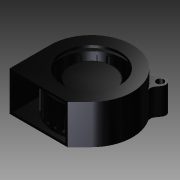
# Autodesk Inventor part: FanRadial40mm
Saved by Autodesk Inventor 2015 (Build 190159000, 159)
## iProperties
Created: 2014-12-06
Part Number: FanRadial40mm
Material: ABS Plastic
Document SubType Name: Modeling
Designer: Jack
Density: 1.06 g/cm^3
Appearance: Smooth - Black
Author: Jack
Autodesk Inventor part; units mm, degrees
ref_plane "YZ Plane" through (0, 0, 0) normal (1, 0, 0) x (0, 1, 0)
ref_plane "XZ Plane" through (0, 0, 0) normal (0, 1, 0) x (-1, 0, 0)
ref_plane "XY Plane" through (0, 0, 0) normal (0, 0, 1) x (1, 0, 0)
sketch "Sketch1" plane through (0, 0, 0) normal (0, 0, 1) x (1, 0, 0)
  arc A0 (14.2809, -14.002) -> (-20, 0) centre (0, 0) ccw
  line L0 (-20, 0) -> (-20, -20)
  line L1 (-20, -20) -> (8.4, -20)
  line L2 (8.4, -20) -> (14.2809, -14.002)
  dimension "d0" = 40
  dimension "d1" = 28.4
  constraints: 6 end point, 3 tangent, 2 point on circle, 1 centre point, 1 coincident, 1 perpendicular, 1 vertical
  measures "d0" diameter of A0
  measures "d1" distance of L0.end L1.end
extrude "Extrusion1" add sketch "Sketch1" along normal blind 19.2
shell "Shell1" thickness 1.2 removed faces 0
sketch "Sketch2" plane through (-20, -20, 0) normal (0, -1, 0) x (1, 0, 0)
  line L0 (1.2, 18) -> (27.896, 18) projected
  line L1 (1.2, 1.2) -> (1.2, 18) projected
  line L2 (27.896, 1.2) -> (1.2, 1.2) projected
  line L3 (27.896, 1.2) -> (27.896, 18) projected
  point P0 (20, 0)
extrude "Extrusion2" cut sketch "Sketch2" against normal blind 2
sketch "Sketch3" plane through (-18.8, -20, 1.2) normal (0, 0, 1) x (1, 0, 0)
  line L0 (26.696, 0) -> (0, 0) projected
  line L1 (26.696, 0) -> (26.696, 1.2) projected
  line L2 (32.224, 6.8381) -> (26.696, 1.2) projected
  line L3 (26.696, 1.2) -> (25.5194, 0)
  constraints: 2 end point, 1 collinear, 1 point on line
extrude "Extrusion3" add sketch "Sketch3" along normal up to next
sketch "Sketch4" plane through (0, 0, 0) normal (0, 0, -1) x (-1, 0, 0)
  arc A0 (20, 0) -> (-14.2809, -14.002) centre (0, 0) ccw projected
  line L0 (-14.2809, -14.002) -> (-8.4, -20) projected
  line L1 (-8.4, -20) -> (20, -20) projected
  circle A1 centre (18.9, 17.5) radius 1.75
  circle A2 centre (-16.1, 17.5) radius 1.75
  circle A3 centre (-16.1, -17.5) radius 1.75
  circle A4 centre (-16.1, 17.5) radius 2.75
  circle A5 centre (18.9, 17.5) radius 2.75
  circle A6 centre (-16.1, -17.5) radius 2.75
  line L2 (21.1527, 15.9227) -> (17.1769, 10.2447)
  arc A7 (20, 0) -> (-14.2809, -14.002) centre (0, 0) ccw projected
  line L3 (17.3227, 19.7527) -> (11.9823, 16.0133)
  line L4 (-14.5227, 19.7527) -> (-10.5652, 16.9816)
  line L5 (-18.3527, 15.9227) -> (-15.7945, 12.2692)
  line L6 (-14.5227, -19.7527) -> (-11.0361, -17.3114)
  line L7 (-16.1, -17.5) -> (18.9, 17.5) construction
  line L8 (-16.1, 17.5) -> (1.4, 0) construction
  line L9 (-18.3527, -15.9227) -> (-15.7945, -12.2692)
  dimension "d9" = 35
  dimension "d10" = 35
  dimension "d11" = 3.5
  dimension "d12" = 5.5
  dimension "d17" = 2.5
  dimension "d18" = 7.7
  dimension "d19" = 10
  dimension "d20" = 10
  dimension "d21" = 10
  dimension "d22" = 10
  dimension "d23" = 10
  dimension "d24" = 10
  constraints: 16 end point, 16 point on circle, 6 centre point, 6 tangent, 4 equal radius, 3 coincident, 1 horizontal alignment, 1 midpoint, 1 perpendicular, 1 point on line, 1 vertical alignment
  measures "d9" distance of A1.centre A2.centre
  measures "d10" distance of A3.centre A2.centre
  measures "d11" diameter of A2
  measures "d12" diameter of A4
  measures "d17" distance from line of L1 A3.centre
  measures "d18" horizontal distance of L0.end A3.centre
  measures "d19" angle of L7 L9
  measures "d20" angle of L7 L6
  measures "d21" angle of L7 L3
  measures "d22" angle of L7 L2
  measures "d23" angle of L8 L5
  measures "d24" angle of L8 L4
extrude "Extrusion4" add sketch "Sketch4" against normal blind 13
fillet "Fillet1" radius 3 6 edges at (15.7945, -12.2692, 6.5) (11.0361, -17.3114, 6.5) (15.7945, 12.2692, 6.5) (10.5652, 16.9816, 6.5) (-11.9823, 16.0133, 6.5) (-17.1769, 10.2447, 6.5)
sketch "Sketch5" plane through (0, 0, 19.2) normal (0, 0, 1) x (1, 0, 0)
  arc A0 (14.2809, -14.002) -> (-20, 0) centre (0, 0) ccw projected
  circle A1 centre (0, 0) radius 14
  dimension "d28" = 28
  constraints: 1 centre point, 1 coincident
  measures "d28" diameter of A1
extrude "Extrusion5" cut sketch "Sketch5" against normal up to next
sketch "Sketch6" plane through (-18.8, -20, 1.2) normal (0, 0, 1) x (1, 0, 0)
  arc A0 (32.224, 6.8381) -> (0, 20) centre (18.8, 20) ccw projected
  circle A1 centre (18.8, 20) radius 18
  dimension "d31" = 36
  constraints: 1 centre point, 1 coincident
  measures "d31" diameter of A1
extrude "Extrusion6" add sketch "Sketch6" along normal blind 14
sketch "Sketch7" plane through (0, 0, 15.2) normal (0, 0, 1) x (1, 0, 0)
  circle A0 centre (0, 0) radius 18 projected
  circle A1 centre (0, 0) radius 11
  circle A2 centre (0, 0) radius 16
  dimension "d34" = 22
  dimension "d35" = 2
  constraints: 2 centre point, 2 coincident
  measures "d34" diameter of A1
  measures "d35" radial gap between concentric circles of A0 A2
extrude "Extrusion7" cut sketch "Sketch7" against normal blind 12.5 contours A2
fillet "Fillet2" radius 1 1 edges at (-11, 0, 15.2)
ref_plane "Work Plane1" through (0, 0, 13.7) normal (0, 0, 1) x (1, 0, 0)
sketch "Sketch8" plane through (0, 0, 13.7) normal (0, 0, 1) x (1, 0, 0)
  circle A0 centre (0, 0) radius 18 projected
  circle A1 centre (0, 0) radius 16 projected
  circle A2 centre (0, 0) radius 16 projected
  line L0 (-0.7111, -15.9842) -> (-0.8, -17.9822)
  circle A3 centre (0, 0) radius 18 projected
  line L1 (0.7111, -15.9842) -> (0.8, -17.9822)
  dimension "d40" = 1.6
  dimension "d42" = 0.8
  constraints: 8 point on circle, 4 end point, 2 point on line
  measures "d40" distance of L1.end L0.end
  measures "d42" horizontal distance of point (0, 0) L1.end
extrude "Extrusion8" cut sketch "Sketch8" against normal blind 11 contours L0 A1 L1 A0 picked at (0.079, -17.3314)
pattern_circular "Circular Pattern1" count 30 over 360 about axis through (0, 0, 15.2) along (0, 0, -1) of "Extrusion8"
sketch "Sketch9" plane through (-20, -20, 0) normal (0, -1, 0) x (1, 0, 0)
  line L0 (26.7194, 1.2) -> (26.7194, 18) projected
  line L1 (1.2, 1.2) -> (1.2, 18) projected
  line L2 (26.7194, 18) -> (27.2, 18)
  line L3 (26.7194, 18) -> (33.424, 18) projected
  line L4 (27.2, 18) -> (27.2, 1.2)
  line L5 (33.424, 1.2) -> (26.7194, 1.2) projected
  line L6 (26.7194, 1.2) -> (27.2, 1.2)
  point P0 (20, 0)
  dimension "d48" = 26
  constraints: 6 end point, 2 point on line, 1 collinear, 1 perpendicular
  measures "d48" distance between parallel lines of L1 L4
extrude "Extrusion9" cut sketch "Sketch9" against normal blind 0.75
sketch "Sketch10" plane through (0, 0, 13) normal (0, 0, 1) x (1, 0, 0)
  circle A0 centre (16.1, -17.5) radius 1.75 projected
  arc A1 (14.2809, -14.002) -> (16.9178, -10.6672) centre (0, 0) ccw projected
  line L0 (9.2561, -19.1269) -> (14.2809, -14.002) projected
  arc A2 (13.1189, -18.7697) -> (9.2561, -19.1269) centre (11.3982, -21.2272) ccw projected
  line L1 (13.1189, -18.7697) -> (14.5227, -19.7527) projected
  arc A3 (14.5227, -19.7527) -> (18.3527, -15.9227) centre (16.1, -17.5) ccw projected
  line L2 (18.3527, -15.9227) -> (16.998, -13.988) projected
  arc A4 (16.9178, -10.6672) -> (16.998, -13.988) centre (19.4554, -12.2673) ccw projected
extrude "Extrusion10" cut sketch "Sketch10" against normal up to next
body "Solid1"
